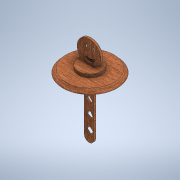
# Autodesk Inventor part: PalitoPaleta
Saved by Autodesk Inventor 2021 (Build 250183000, 183)
## iProperties
Created: 2021-03-05
Part Number: PalitoPaleta
Material: Polypropylene
Document SubType Name: Modeling
Designer: uriel
Density: 0.899 g/cm^3
Appearance: English Oak
Author: uriel
Autodesk Inventor part; units mm, degrees
ref_plane "YZ Plane" through (0, 0, 0) normal (1, 0, 0) x (0, 1, 0)
ref_plane "XZ Plane" through (0, 0, 0) normal (0, 1, 0) x (-1, 0, 0)
ref_plane "XY Plane" through (0, 0, 0) normal (0, 0, 1) x (1, 0, 0)
sketch "Sketch1" plane through (0, 0, 0) normal (0, 0, 1) x (1, 0, 0)
  line L0 (5, 0) -> (5, -70)
  line L1 (5, -70) -> (-5, -70)
  line L2 (-5, -70) -> (-5, 0)
  arc A0 (5, 0) -> (-5, 0) centre (0, 11.4564) ccw
  point P0 (0, 0)
  dimension "d0" = 70
  dimension "d1" = 12.5
  dimension "d2" = 10
  dimension "d3" = 5
  dimension "d4" = 70
  constraints: 6 end point, 2 parallel, 2 point on circle, 1 centre point, 1 horizontal, 1 vertical
  measures "d0" distance of L0.start L0.end
  measures "d1" radius of A0
  measures "d2" distance of L0.end L1.end
  measures "d3" distance from line of L0 point (0, 0)
  measures "d4" distance from line of point (0, 0) L1
extrude "Extrusion1" add sketch "Sketch1" along normal mid plane 2
sketch "Sketch2" plane through (0, 0, 0) normal (0, 1, 0) x (-1, 0, 0)
  point P0 (0, 0)
sketch "Sketch3" plane through (0, 0, 0) normal (1, 0, 0) x (0, 1, 0)
  line L0 (0, 0) -> (0, -12)
  line L1 (0, -12) -> (-3.5872, -12)
  line L2 (-3.5872, -12) -> (-3.5872, -25)
  line L3 (-3.5872, -25) -> (-7.267, -28.2855)
  line L4 (-7.267, -28.2855) -> (-3.5872, 0)
  line L5 (-3.5872, 0) -> (0, 0)
  line L6 (0, 1) -> (0, -1) projected
  dimension "d7" = 12
  dimension "d8" = 13
  constraints: 12 end point, 3 perpendicular, 1 point on line, 1 vertical
  measures "d7" distance of L0.start L0.end
  measures "d8" distance of L1.end L2.end
revolve "Revolution1" add sketch "Sketch3" angle 360 about axis through (0, -3.5872, 0) along (0, 1, 0) separate body
shell "Shell1" thickness 1 removed faces 1 at (0, -6.4493, 21.9999) bodies 2
fillet "Fillet1" radius 5 2 edges at (-5, -70, 0) (5, -70, 0)
sketch "Sketch4" plane through (0, 0, -1) normal (0, 0, -1) x (-1, 0, 0)
  line L0 (2.2552, -11.8066) -> (-2.2764, -11.7698)
  line L1 (-2.2764, -11.7698) -> (0.0213, -7.8637)
  line L2 (0.0213, -7.8637) -> (2.2552, -11.8066)
  line L3 (-0.1086, -23.8401) -> (-3.133, -18.5019)
  line L4 (-3.133, -18.5019) -> (3.0022, -18.5517)
  line L5 (3.0022, -18.5517) -> (-0.1086, -23.8401)
  line L6 (-0.1941, -34.3618) -> (-3.4609, -31.0414)
  line L7 (-3.4609, -31.0414) -> (-0.1405, -27.7746)
  line L8 (-0.1405, -27.7746) -> (3.1263, -31.095)
  line L9 (3.1263, -31.095) -> (-0.1941, -34.3618)
  line L10 (-1.1276, -48.1608) -> (-3.9272, -44.8911)
  line L11 (-3.9272, -44.8911) -> (-1.6827, -41.2181)
  line L12 (-1.6827, -41.2181) -> (2.5041, -42.2177)
  line L13 (2.5041, -42.2177) -> (2.8472, -46.5086)
  line L14 (2.8472, -46.5086) -> (-1.1276, -48.1608)
  line L15 (0.4107, -62.7603) -> (-3.2306, -61.5876)
  line L16 (-3.2306, -61.5876) -> (-4.0358, -57.8478)
  line L17 (-4.0358, -57.8478) -> (-1.1995, -55.2806)
  line L18 (-1.1995, -55.2806) -> (2.4418, -56.4532)
  line L19 (2.4418, -56.4532) -> (3.247, -60.1931)
  line L20 (3.247, -60.1931) -> (0.4107, -62.7603)
  point P0 (0, 0)
  point P1 (0, -10.48)
  point P2 (-0.0798, -20.2979)
  point P3 (-0.1673, -31.0682)
  point P4 (-0.2772, -44.5992)
  point P5 (-0.3944, -59.0204)
  constraints: 42 end point, 47 other
extrude "Extrusion2" cut sketch "Sketch4" along normal through all both and the other way through all bodies 1
combine bodies "Combine1" operation type add bodies to combine 1 2
sketch "Sketch5" plane through (0, 0, 0) normal (0, 0, 1) x (1, 0, 0)
  arc A0 (-6.4273, 8.502) -> (6.4273, 8.502) centre (0, 8.502) ccw
  line L0 (0, 8.502) -> (6.4273, 8.502)
  line L1 (6.4273, 8.502) -> (0, 8.502)
  line L2 (-6.4273, 8.502) -> (0, 8.502)
  arc A1 (-6.4273, 8.502) -> (6.4273, 8.502) centre (0, 17.3006) ccw
  ellipse E0 centre (4.567, 15.0845) end of major axis (4.567, 18.1799) minor radius 1.9384
  ellipse E1 centre (-3.7905, 15.0845) end of major axis (-3.7905, 18.1799) minor radius 1.6366
  point P0 (0, 0)
  constraints: 6 end point, 4 point on circle, 2 centre point, 1 collinear, 1 horizontal, 1 point on line, 4 other
extrude "Extrusion3" cut sketch "Sketch5" along normal mid plane 3 contours A1 A0 | E0 | E1 bodies 1
equation "\"d3\" = 0.5 * d2"
equation "\"d4\" = d0"
body "Solid1"
